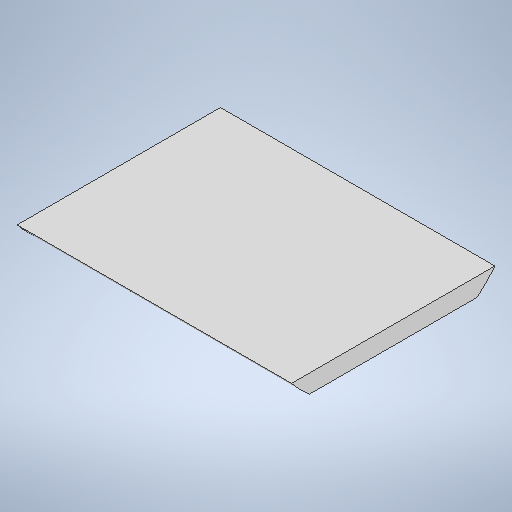
# Autodesk Inventor part: Base
Saved by Autodesk Inventor 2025.3 (Build 293356000, 356)
## iProperties
Created: 2025-05-16
Part Number: Base
Material: Generic
Document SubType Name: Modeling
Designer: Verðandi
Density: 1 g/cm^3
Appearance: Default
Author: Verðandi
Autodesk Inventor part; units mm, degrees
ref_plane "YZ Plane" through (0, 0, 0) normal (1, 0, 0) x (0, 1, 0)
ref_plane "XZ Plane" through (0, 0, 0) normal (0, 1, 0) x (-1, 0, 0)
ref_plane "XY Plane" through (0, 0, 0) normal (0, 0, 1) x (1, 0, 0)
sketch "Sketch1" plane through (0, 0, 0) normal (1, 0, 0) x (0, 1, 0)
  circle A0 centre (0, 0) radius 71
  dimension "d0" = 142
  constraints: 1 centre point, 1 coincident
  measures "d0" diameter of A0
extrude "Extrusion1" add sketch "Sketch1" along normal blind 150
sketch "Sketch2" plane through (150, 0, 0) normal (1, 0, 0) x (0, 0, -1)
  line L0 (0, 0) -> (0, -44.2)
  circle A0 centre (0, 0) radius 71 projected
  line L1 (-55.564, -44.2) -> (55.564, -44.2)
  dimension "d3" = 44.2
  constraints: 4 end point, 2 point on circle, 1 horizontal, 1 vertical
  measures "d3" distance of L0.start L0.end
extrude "Extrusion2" cut sketch "Sketch2" against normal blind 150 contours A0 L1 picked at (-0.2063, 32.437)
sketch "Sketch3" plane through (150, 0, 0) normal (1, 0, 0) x (0, 0, -1)
  line L0 (0, 0) -> (0, -54.2)
  arc A0 (-55.564, -44.2) -> (55.564, -44.2) centre (0, 0) ccw projected
  line L1 (-45.8624, -54.2) -> (45.8624, -54.2)
  dimension "d6" = 54.2
  constraints: 4 end point, 2 point on circle, 1 horizontal, 1 vertical
  measures "d6" distance of L0.start L0.end
extrude "Extrusion3" cut sketch "Sketch3" against normal blind 150
body "Solid1"
